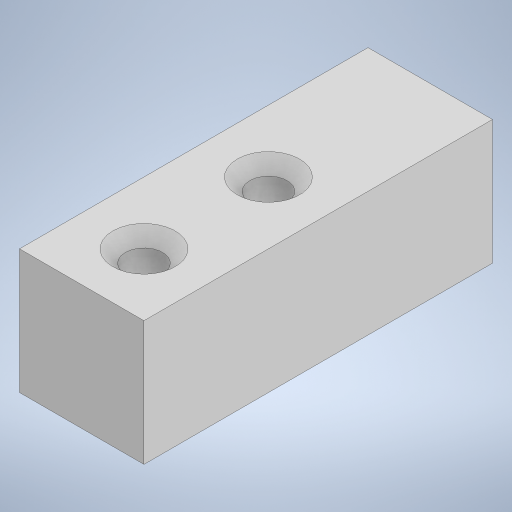
# Autodesk Inventor part: Ограничитель
Saved by Autodesk Inventor 2023 (Build 270158000, 158)
## iProperties
Created: 2022-05-17
Part Number: Ограничитель
Material: Типовые
Document SubType Name: Modeling
Designer: avkap
Density: 1 g/cm^3
Appearance: По умолчанию
Author: avkap
Autodesk Inventor part; units mm, degrees
ref_plane "YZ Plane" through (0, 0, 0) normal (1, 0, 0) x (0, 1, 0)
ref_plane "XZ Plane" through (0, 0, 0) normal (0, 1, 0) x (-1, 0, 0)
ref_plane "XY Plane" through (0, 0, 0) normal (0, 0, 1) x (1, 0, 0)
sketch "Эскиз1" plane through (0, 0, 0) normal (0, 1, 0) x (-1, 0, 0)
  line L0 (0, 0) -> (-10, 0)
  line L1 (-10, 0) -> (-10, -28)
  line L2 (-10, -28) -> (0, -28)
  line L3 (0, -28) -> (0, 0)
  line L4 (-5, 0) -> (-5, -10)
  line L5 (-5, -10) -> (-5, -20)
  line L6 (-5, -20) -> (-5, -15)
  line L7 (-5, 0) -> (-5, -5)
  circle A0 centre (-5, -5) radius 1.5
  circle A1 centre (-5, -15) radius 1.5
  dimension "d0" = 10
  dimension "d1" = 28
  dimension "d2" = 10
  dimension "d3" = 10
  dimension "d4" = 3
  constraints: 16 end point, 3 midpoint, 2 centre point, 2 coincident, 2 parallel, 1 horizontal, 1 perpendicular, 1 point on line, 1 vertical
  measures "d0" distance of L2.end L1.end
  measures "d1" distance of L1.end L0.end
  measures "d2" distance of L4.start L4.end
  measures "d3" distance of L4.end L5.end
  measures "d4" diameter of A0
extrude "Выдавливание1" add sketch "Эскиз1" along normal blind 10
chamfer "Фаска1" distance 1 angle 45 4 edges at (6.5, 10, -5) (6.5, 10, -15) (6.5, 0, -15) (6.5, 0, -5)
